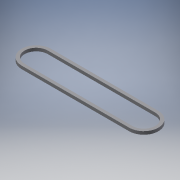
# Autodesk Inventor part: ketting1
Saved by Autodesk Inventor 2017 (Build 210142000, 142)
## iProperties
Created: 2017-02-19
Part Number: ketting1
Material: Generic
Document SubType Name: Modeling
Designer: user
Density: 1 g/cm^3
Appearance: Default
Author: user
Autodesk Inventor part; units mm, degrees
ref_plane "YZ Plane" through (0, 0, 0) normal (1, 0, 0) x (0, 1, 0)
ref_plane "XZ Plane" through (0, 0, 0) normal (0, 1, 0) x (-1, 0, 0)
ref_plane "XY Plane" through (0, 0, 0) normal (0, 0, 1) x (1, 0, 0)
sketch "Sketch1" plane through (0, 0, 0) normal (0, 0, 1) x (1, 0, 0)
  circle A0 centre (0, 0) radius 10 projected
  circle A1 centre (0, 0) radius 30 projected
  circle A2 centre (400, 0) radius 10 projected
  circle A3 centre (400, 0) radius 30 projected
  line L0 (0, 38) -> (400, 38)
  arc A4 (400, -38) -> (400, 38) centre (400, 0) ccw
  line L1 (400, -38) -> (0, -38)
  arc A5 (0, 38) -> (0, -38) centre (0, 0) ccw
  line L2 (400, 30) -> (0, 30)
  arc A6 (0, 30) -> (0, -30) centre (0, 0) ccw
  line L3 (0, -30) -> (400, -30)
  arc A7 (400, -30) -> (400, 30) centre (400, 0) ccw
  dimension "d0" = 8
  constraints: 8 end point, 8 point on circle, 5 tangent, 4 centre point, 2 parallel, 1 coincident, 1 concentric, 1 horizontal, 3 other
  measures "d0" distance between parallel lines of L0 L2
extrude "Extrusion1" add sketch "Sketch1" against normal blind 8 contours L0 A4 L1 A5
body "Solid1"
